Autodesk Inventor part; units mm, degrees
(part 2 of 2)
  spline S141 degree 2 poles (-52.2442, -8.1666) (-52.2404, -7.8589) (-52.0134, -7.5935) (-51.8404, -7.5974) knots 0 0 0 1 2 2 2
  spline S142 degree 2 poles (-51.8404, -7.5974) (-51.675, -7.5935) (-51.4904, -7.8474) (-51.4904, -8.1358) knots 0 0 0 1 2 2 2
  line L206 (-51.4904, -8.1358) -> (-51.4904, -9.6935)
  line L207 (-51.4904, -9.6935) -> (-50.198, -9.6935)
  line L208 (-50.198, -9.6935) -> (-50.198, -8.1666)
  spline S143 degree 2 poles (-50.198, -8.1666) (-50.1942, -7.8589) (-49.9711, -7.5935) (-49.7942, -7.5974) knots 0 0 0 1 2 2 2
  spline S144 degree 2 poles (-49.7942, -7.5974) (-49.6404, -7.5935) (-49.448, -7.8474) (-49.448, -8.1358) knots 0 0 0 1 2 2 2
  line L209 (-49.448, -8.1358) -> (-49.448, -9.6935)
  line L210 (-49.448, -9.6935) -> (-48.1557, -9.6935)
  line L211 (-48.1557, -9.6935) -> (-48.1557, -7.9127)
  spline S145 degree 2 poles (-48.1557, -7.9127) (-48.1596, -7.4204) (-48.4827, -6.8051) (-49.0442, -6.5127) (-49.4019, -6.5127) knots 0 0 0 1 2 3 3 3
  spline S146 degree 2 poles (-45.9442, -9.7512) (-45.4096, -9.7474) (-44.5942, -9.3358) (-44.1327, -8.6089) (-44.1288, -8.1281) knots 0 0 0 1 2 3 3 3
  spline S147 degree 2 poles (-44.1288, -8.1281) (-44.1327, -7.6512) (-44.5942, -6.9243) (-45.4096, -6.5166) (-45.9442, -6.5127) knots 0 0 0 1 2 3 3 3
  spline S148 degree 2 poles (-45.9442, -6.5127) (-46.4788, -6.5166) (-47.2942, -6.9243) (-47.7596, -7.6512) (-47.7634, -8.1281) knots 0 0 0 1 2 3 3 3
  spline S149 degree 2 poles (-47.7634, -8.1281) (-47.7596, -8.6089) (-47.2942, -9.3358) (-46.4788, -9.7474) (-45.9442, -9.7512) knots 0 0 0 1 2 3 3 3
  spline S150 degree 2 poles (-45.9442, -8.7474) (-46.1673, -8.7474) (-46.4519, -8.4358) (-46.4557, -8.1281) knots 0 0 0 1 2 2 2
  spline S151 degree 2 poles (-46.4557, -8.1281) (-46.4519, -7.8243) (-46.1673, -7.5166) (-45.9442, -7.5166) knots 0 0 0 1 2 2 2
  spline S152 degree 2 poles (-45.9442, -7.5166) (-45.725, -7.5166) (-45.4404, -7.8243) (-45.4365, -8.1281) knots 0 0 0 1 2 2 2
  spline S153 degree 2 poles (-45.4365, -8.1281) (-45.4404, -8.4358) (-45.725, -8.7474) (-45.9442, -8.7474) knots 0 0 0 1 2 2 2
  spline S154 degree 2 poles (-40.4865, -7.6051) (-40.2134, -7.4666) (-39.9327, -7.0204) (-39.9327, -6.7397) knots 0 0 0 1 2 2 2
  spline S155 degree 2 poles (-39.9327, -6.7397) (-39.9288, -6.2743) (-40.725, -5.7012) (-41.548, -5.6935) knots 0 0 0 1 2 2 2
  line L212 (-41.548, -5.6935) -> (-43.6865, -5.6935)
  line L213 (-43.6865, -5.6935) -> (-43.6865, -9.6935)
  line L214 (-43.6865, -9.6935) -> (-41.4327, -9.6935)
  spline S156 degree 2 poles (-41.4327, -9.6935) (-40.6057, -9.6897) (-39.748, -9.1166) (-39.7442, -8.5935) knots 0 0 0 1 2 2 2
  spline S157 degree 2 poles (-39.7442, -8.5935) (-39.748, -8.2358) (-40.1327, -7.732) (-40.4865, -7.6051) knots 0 0 0 1 2 2 2
  line L215 (-41.548, -8.7512) -> (-42.3596, -8.7512)
  line L216 (-42.3596, -8.7512) -> (-42.3596, -8.1243)
  line L217 (-42.3596, -8.1243) -> (-41.548, -8.1243)
  spline S158 degree 2 poles (-41.548, -8.1243) (-41.325, -8.1243) (-41.1019, -8.282) (-41.1019, -8.4358) knots 0 0 0 1 2 2 2
  spline S159 degree 2 poles (-41.1019, -8.4358) (-41.1019, -8.5935) (-41.325, -8.7512) (-41.548, -8.7512) knots 0 0 0 1 2 2 2
  spline S160 degree 2 poles (-41.7327, -6.6358) (-41.5057, -6.6358) (-41.2904, -6.7858) (-41.2904, -6.9358) knots 0 0 0 1 2 2 2
  spline S161 degree 2 poles (-41.2904, -6.9358) (-41.2904, -7.082) (-41.5057, -7.232) (-41.7327, -7.232) knots 0 0 0 1 2 2 2
  line L218 (-41.7327, -7.232) -> (-42.3596, -7.232)
  line L219 (-42.3596, -7.232) -> (-42.3596, -6.6358)
  line L220 (-42.3596, -6.6358) -> (-41.7327, -6.6358)
  line L221 (-37.1827, -6.5704) -> (-37.1827, -8.0397)
  spline S162 degree 2 poles (-37.1827, -8.0397) (-37.1904, -8.382) (-37.448, -8.6704) (-37.6211, -8.6666) knots 0 0 0 1 2 2 2
  spline S163 degree 2 poles (-37.6211, -8.6666) (-37.8134, -8.6704) (-38.0288, -8.4012) (-38.0288, -8.0743) knots 0 0 0 1 2 2 2
  line L222 (-38.0288, -8.0743) -> (-38.0288, -6.5704)
  line L223 (-38.0288, -6.5704) -> (-39.3211, -6.5704)
  line L224 (-39.3211, -6.5704) -> (-39.3211, -8.2974)
  spline S164 degree 2 poles (-39.3211, -8.2974) (-39.3173, -8.8012) (-38.975, -9.4474) (-38.3827, -9.7512) (-38.0057, -9.7512) knots 0 0 0 1 2 3 3 3
  spline S165 degree 2 poles (-38.0057, -9.7512) (-37.7519, -9.7512) (-37.298, -9.5781) (-37.1211, -9.3974) knots 0 0 0 1 2 2 2
  line L225 (-37.1211, -9.3974) -> (-37.1211, -9.6935)
  line L226 (-37.1211, -9.6935) -> (-35.8904, -9.6935)
  line L227 (-35.8904, -9.6935) -> (-35.8904, -6.5704)
  line L228 (-35.8904, -6.5704) -> (-37.1827, -6.5704)
  line L229 (-33.1557, -5.4551) -> (-33.1557, -6.782)
  spline S166 degree 2 poles (-33.1557, -6.782) (-33.298, -6.6435) (-33.6904, -6.5127) (-33.948, -6.5127) knots 0 0 0 1 2 2 2
  spline S167 degree 2 poles (-33.948, -6.5127) (-34.3634, -6.5166) (-35.0404, -6.9012) (-35.4519, -7.6243) (-35.4557, -8.1281) knots 0 0 0 1 2 3 3 3
  spline S168 degree 2 poles (-35.4557, -8.1281) (-35.4519, -8.632) (-35.0404, -9.3589) (-34.3634, -9.7474) (-33.948, -9.7512) knots 0 0 0 1 2 3 3 3
  spline S169 degree 2 poles (-33.948, -9.7512) (-33.6596, -9.7512) (-33.2327, -9.5974) (-33.0942, -9.4358) knots 0 0 0 1 2 2 2
  line L230 (-33.0942, -9.4358) -> (-33.0942, -9.6935)
  line L231 (-33.0942, -9.6935) -> (-31.8634, -9.6935)
  line L232 (-31.8634, -9.6935) -> (-31.8634, -5.4551)
  line L233 (-31.8634, -5.4551) -> (-33.1557, -5.4551)
  spline S170 degree 2 poles (-33.6404, -8.7435) (-33.8596, -8.7435) (-34.1442, -8.432) (-34.148, -8.1281) knots 0 0 0 1 2 2 2
  spline S171 degree 2 poles (-34.148, -8.1281) (-34.1442, -7.8243) (-33.8596, -7.5166) (-33.6404, -7.5166) knots 0 0 0 1 2 2 2
  spline S172 degree 2 poles (-33.6404, -7.5166) (-33.4211, -7.5166) (-33.1365, -7.8243) (-33.1327, -8.1281) knots 0 0 0 1 2 2 2
  spline S173 degree 2 poles (-33.1327, -8.1281) (-33.1365, -8.432) (-33.4211, -8.7435) (-33.6404, -8.7435) knots 0 0 0 1 2 2 2
  line L234 (-29.1288, -5.4551) -> (-29.1288, -6.782)
  spline S174 degree 2 poles (-29.1288, -6.782) (-29.2711, -6.6435) (-29.6634, -6.5127) (-29.9211, -6.5127) knots 0 0 0 1 2 2 2
  spline S175 degree 2 poles (-29.9211, -6.5127) (-30.3365, -6.5166) (-31.0134, -6.9012) (-31.425, -7.6243) (-31.4288, -8.1281) knots 0 0 0 1 2 3 3 3
  spline S176 degree 2 poles (-31.4288, -8.1281) (-31.425, -8.632) (-31.0134, -9.3589) (-30.3365, -9.7474) (-29.9211, -9.7512) knots 0 0 0 1 2 3 3 3
  spline S177 degree 2 poles (-29.9211, -9.7512) (-29.6327, -9.7512) (-29.2057, -9.5974) (-29.0673, -9.4358) knots 0 0 0 1 2 2 2
  line L235 (-29.0673, -9.4358) -> (-29.0673, -9.6935)
  line L236 (-29.0673, -9.6935) -> (-27.8365, -9.6935)
  line L237 (-27.8365, -9.6935) -> (-27.8365, -5.4551)
  line L238 (-27.8365, -5.4551) -> (-29.1288, -5.4551)
  spline S178 degree 2 poles (-29.6134, -8.7435) (-29.8327, -8.7435) (-30.1173, -8.432) (-30.1211, -8.1281) knots 0 0 0 1 2 2 2
  spline S179 degree 2 poles (-30.1211, -8.1281) (-30.1173, -7.8243) (-29.8327, -7.5166) (-29.6134, -7.5166) knots 0 0 0 1 2 2 2
  spline S180 degree 2 poles (-29.6134, -7.5166) (-29.3942, -7.5166) (-29.1096, -7.8243) (-29.1057, -8.1281) knots 0 0 0 1 2 2 2
  spline S181 degree 2 poles (-29.1057, -8.1281) (-29.1096, -8.432) (-29.3942, -8.7435) (-29.6134, -8.7435) knots 0 0 0 1 2 2 2
  line L239 (-25.0096, -6.5704) -> (-25.6673, -8.2435)
  line L240 (-25.6673, -8.2435) -> (-26.3096, -6.5704)
  line L241 (-26.3096, -6.5704) -> (-27.6365, -6.5704)
  line L242 (-27.6365, -6.5704) -> (-26.3211, -9.7358)
  spline S182 degree 2 poles (-26.3211, -9.7358) (-26.375, -9.7935) (-26.5288, -9.8589) (-26.6442, -9.8589) knots 0 0 0 1 2 2 2
  spline S183 degree 2 poles (-26.6442, -9.8589) (-26.7596, -9.8589) (-27.0019, -9.7704) (-27.098, -9.6974) knots 0 0 0 1 2 2 2
  line L243 (-27.098, -9.6974) -> (-27.5288, -10.5781)
  spline S184 degree 2 poles (-27.5288, -10.5781) (-27.3634, -10.7089) (-26.8442, -10.8589) (-26.5788, -10.8589) knots 0 0 0 1 2 2 2
  spline S185 degree 2 poles (-26.5788, -10.8589) (-26.248, -10.8627) (-25.6942, -10.6627) (-25.2442, -10.182) (-25.0711, -9.7589) knots 0 0 0 1 2 3 3 3
  line L244 (-25.0711, -9.7589) -> (-23.7865, -6.5704)
  line L245 (-23.7865, -6.5704) -> (-25.0096, -6.5704)
  line L246 (24.7318, 2.5001) -> (24.0485, 3.4796)
  spline S186 degree 2 poles (24.0485, 3.4796) (24.3476, 3.6086) (24.6732, 4.0984) (24.6761, 4.4415) knots 0 0 0 1 2 2 2
  spline S187 degree 2 poles (24.6761, 4.4415) (24.6702, 4.9606) (23.9693, 5.5442) (23.3505, 5.5501) knots 0 0 0 1 2 2 2
  line L247 (23.3505, 5.5501) -> (22.0308, 5.5501)
  line L248 (22.0308, 5.5501) -> (22.0308, 2.5001)
  line L249 (22.0308, 2.5001) -> (22.7376, 2.5001)
  line L250 (22.7376, 2.5001) -> (22.7376, 3.3476)
  line L251 (22.7376, 3.3476) -> (23.3505, 3.3476)
  line L252 (23.3505, 3.3476) -> (23.3857, 3.3476)
  line L253 (23.3857, 3.3476) -> (23.9752, 2.5001)
  line L254 (23.9752, 2.5001) -> (24.7318, 2.5001)
  spline S188 degree 2 poles (23.9605, 4.4415) (23.9605, 4.1923) (23.635, 3.9136) (23.3124, 3.9107) knots 0 0 0 1 2 2 2
  line L255 (23.3124, 3.9107) -> (22.7376, 3.9107)
  line L256 (22.7376, 3.9107) -> (22.7376, 4.9753)
  line L257 (22.7376, 4.9753) -> (23.3124, 4.9753)
  spline S189 degree 2 poles (23.3124, 4.9753) (23.635, 4.9724) (23.9605, 4.6967) (23.9605, 4.4415) knots 0 0 0 1 2 2 2
  line L258 (26.8639, 4.8433) -> (26.8639, 3.682)
  spline S190 degree 2 poles (26.8639, 3.682) (26.8609, 3.3594) (26.5647, 3.0514) (26.3243, 3.0514) knots 0 0 0 1 2 2 2
  spline S191 degree 2 poles (26.3243, 3.0514) (26.0955, 3.0485) (25.8492, 3.3242) (25.8492, 3.6174) knots 0 0 0 1 2 2 2
  line L259 (25.8492, 3.6174) -> (25.8492, 4.8433)
  line L260 (25.8492, 4.8433) -> (25.1688, 4.8433)
  line L261 (25.1688, 4.8433) -> (25.1688, 3.5177)
  spline S192 degree 2 poles (25.1688, 3.5177) (25.1717, 3.157) (25.4239, 2.6907) (25.8756, 2.4649) (26.1718, 2.4649) knots 0 0 0 1 2 3 3 3
  spline S193 degree 2 poles (26.1718, 2.4649) (26.3888, 2.4649) (26.7642, 2.6233) (26.8991, 2.7787) knots 0 0 0 1 2 2 2
  line L262 (26.8991, 2.7787) -> (26.8991, 2.5001)
  line L263 (26.8991, 2.5001) -> (27.5443, 2.5001)
  line L264 (27.5443, 2.5001) -> (27.5443, 4.8433)
  line L265 (27.5443, 4.8433) -> (26.8639, 4.8433)
  spline S194 degree 2 poles (29.6001, 4.8785) (29.3596, 4.8785) (28.9637, 4.7201) (28.8229, 4.5706) knots 0 0 0 1 2 2 2
  line L266 (28.8229, 4.5706) -> (28.8229, 4.8433)
  line L267 (28.8229, 4.8433) -> (28.1748, 4.8433)
  line L268 (28.1748, 4.8433) -> (28.1748, 2.5001)
  line L269 (28.1748, 2.5001) -> (28.8552, 2.5001)
  line L270 (28.8552, 2.5001) -> (28.8552, 3.6585)
  spline S195 degree 2 poles (28.8552, 3.6585) (28.8581, 3.9811) (29.166, 4.292) (29.4153, 4.292) knots 0 0 0 1 2 2 2
  spline S196 degree 2 poles (29.4153, 4.292) (29.6441, 4.292) (29.8904, 4.0222) (29.8904, 3.7377) knots 0 0 0 1 2 2 2
  line L271 (29.8904, 3.7377) -> (29.8904, 2.5001)
  line L272 (29.8904, 2.5001) -> (30.5708, 2.5001)
  line L273 (30.5708, 2.5001) -> (30.5708, 3.8433)
  spline S197 degree 2 poles (30.5708, 3.8433) (30.5679, 4.1981) (30.3157, 4.6586) (29.8787, 4.8785) (29.6001, 4.8785) knots 0 0 0 1 2 3 3 3
  line L274 (23.3505, 14.5501) -> (22.0308, 14.5501)
  line L275 (22.0308, 14.5501) -> (22.0308, 11.5001)
  line L276 (22.0308, 11.5001) -> (22.7376, 11.5001)
  line L277 (22.7376, 11.5001) -> (22.7376, 12.3418)
  line L278 (22.7376, 12.3418) -> (23.3505, 12.3418)
  spline S198 degree 2 poles (23.3505, 12.3418) (23.9693, 12.3476) (24.6702, 12.9283) (24.6761, 13.4445) knots 0 0 0 1 2 2 2
  spline S199 degree 2 poles (24.6761, 13.4445) (24.6702, 13.9606) (23.9693, 14.5442) (23.3505, 14.5501) knots 0 0 0 1 2 2 2
  line L279 (23.3124, 12.9166) -> (22.7376, 12.9166)
  line L280 (22.7376, 12.9166) -> (22.7376, 13.9753)
  line L281 (22.7376, 13.9753) -> (23.3124, 13.9753)
  spline S200 degree 2 poles (23.3124, 13.9753) (23.635, 13.9724) (23.9605, 13.6967) (23.9605, 13.4445) knots 0 0 0 1 2 2 2
  spline S201 degree 2 poles (23.9605, 13.4445) (23.9605, 13.1923) (23.635, 12.9195) (23.3124, 12.9166) knots 0 0 0 1 2 2 2
  spline S202 degree 2 poles (26.2861, 11.4649) (26.6615, 11.4678) (27.2393, 11.7728) (27.5677, 12.3154) (27.5707, 12.6732) knots 0 0 0 1 2 3 3 3
  spline S203 degree 2 poles (27.5707, 12.6732) (27.5677, 13.028) (27.2393, 13.5706) (26.6615, 13.8756) (26.2861, 13.8785) knots 0 0 0 1 2 3 3 3
  spline S204 degree 2 poles (26.2861, 13.8785) (25.9107, 13.8756) (25.3301, 13.5706) (24.9987, 13.028) (24.9957, 12.6732) knots 0 0 0 1 2 3 3 3
  spline S205 degree 2 poles (24.9957, 12.6732) (24.9987, 12.3154) (25.3301, 11.7728) (25.9107, 11.4678) (26.2861, 11.4649) knots 0 0 0 1 2 3 3 3
  spline S206 degree 2 poles (26.2861, 12.0221) (26.0251, 12.025) (25.6908, 12.3652) (25.6849, 12.6732) knots 0 0 0 1 2 2 2
  spline S207 degree 2 poles (25.6849, 12.6732) (25.6908, 12.9782) (26.0251, 13.3184) (26.2861, 13.3213) knots 0 0 0 1 2 2 2
  spline S208 degree 2 poles (26.2861, 13.3213) (26.5442, 13.3184) (26.8756, 12.9782) (26.8815, 12.6732) knots 0 0 0 1 2 2 2
  spline S209 degree 2 poles (26.8815, 12.6732) (26.8756, 12.3652) (26.5442, 12.025) (26.2861, 12.0221) knots 0 0 0 1 2 2 2
  line L282 (31.1867, 13.8433) -> (30.6148, 12.2567)
  line L283 (30.6148, 12.2567) -> (30.0576, 13.8433)
  line L284 (30.0576, 13.8433) -> (29.4828, 13.8433)
  line L285 (29.4828, 13.8433) -> (28.908, 12.2567)
  line L286 (28.908, 12.2567) -> (28.3537, 13.8433)
  line L287 (28.3537, 13.8433) -> (27.7144, 13.8433)
  line L288 (27.7144, 13.8433) -> (28.559, 11.5001)
  line L289 (28.559, 11.5001) -> (29.213, 11.5001)
  line L290 (29.213, 11.5001) -> (29.7584, 12.9547)
  line L291 (29.7584, 12.9547) -> (30.2834, 11.5001)
  line L292 (30.2834, 11.5001) -> (30.9374, 11.5001)
  line L293 (30.9374, 11.5001) -> (31.7879, 13.8433)
  line L294 (31.7879, 13.8433) -> (31.1867, 13.8433)
  spline S210 degree 2 poles (34.4009, 12.6614) (34.398, 13.0427) (34.0783, 13.5852) (33.5299, 13.8756) (33.1809, 13.8785) knots 0 0 0 1 2 3 3 3
  spline S211 degree 2 poles (33.1809, 13.8785) (32.8202, 13.8756) (32.26, 13.5676) (31.9345, 13.0251) (31.9316, 12.6702) knots 0 0 0 1 2 3 3 3
  spline S212 degree 2 poles (31.9316, 12.6702) (31.9345, 12.3212) (32.263, 11.7787) (32.8612, 11.4678) (33.2689, 11.4649) knots 0 0 0 1 2 3 3 3
  spline S213 degree 2 poles (33.2689, 11.4649) (33.5856, 11.4649) (34.0724, 11.6585) (34.2367, 11.8432) knots 0 0 0 1 2 2 2
  line L295 (34.2367, 11.8432) -> (33.873, 12.2362)
  spline S214 degree 2 poles (33.873, 12.2362) (33.7557, 12.1218) (33.4712, 12.0104) (33.2865, 12.0104) knots 0 0 0 1 2 2 2
  spline S215 degree 2 poles (33.2865, 12.0104) (33.0167, 12.0133) (32.6677, 12.2597) (32.6149, 12.4796) knots 0 0 0 1 2 2 2
  line L296 (32.6149, 12.4796) -> (34.3862, 12.4796)
  spline S216 degree 2 poles (34.3862, 12.4796) (34.3921, 12.5236) (34.4009, 12.6233) (34.4009, 12.6614) knots 0 0 0 1 2 2 2
  spline S217 degree 2 poles (33.1868, 13.3653) (33.4184, 13.3624) (33.7205, 13.1013) (33.7616, 12.8755) knots 0 0 0 1 2 2 2
  line L297 (33.7616, 12.8755) -> (32.6061, 12.8755)
  spline S218 degree 2 poles (32.6061, 12.8755) (32.6442, 13.1043) (32.9521, 13.3624) (33.1868, 13.3653) knots 0 0 0 1 2 2 2
  line L298 (35.5007, 13.5354) -> (35.5007, 13.8433)
  line L299 (35.5007, 13.8433) -> (34.8525, 13.8433)
  line L300 (34.8525, 13.8433) -> (34.8525, 11.5001)
  line L301 (34.8525, 11.5001) -> (35.5329, 11.5001)
  line L302 (35.5329, 11.5001) -> (35.5329, 12.6057)
  spline S219 degree 2 poles (35.5329, 12.6057) (35.5358, 12.943) (35.8702, 13.2597) (36.1546, 13.2597) knots 0 0 0 1 2 2 2
  spline S220 degree 2 poles (36.1546, 13.2597) (36.1928, 13.2597) (36.2661, 13.2538) (36.3071, 13.2509) knots 0 0 0 1 2 2 2
  line L303 (36.3071, 13.2509) -> (36.3071, 13.8785)
  spline S221 degree 2 poles (36.3071, 13.8785) (36.0344, 13.8785) (35.6268, 13.7055) (35.5007, 13.5354) knots 0 0 0 1 2 2 2
  point P0 (0, 0)
  point P1 (-52.241, -25.46)
  point P2 (-12.021, -25.46)
  point P3 (-56.021, -25.46)
  point P4 (-68.241, -25.46)
  dimension "d70" = 4
  dimension "d71" = 1
  dimension "d72" = 0.4
  dimension "d75" = 5
  constraints: 60 end point, 18 horizontal, 15 vertical alignment, 10 parallel, 8 point on line, 6 collinear, 6 midpoint, 6 perpendicular, 2 coincident, 1 vertical, 4 other
  measures "d70" distance of L1.start L0.start
  measures "d71" distance between parallel lines of L19 L17
  measures "d72" distance between parallel lines of L17 L7
  measures "d75" distance of L43.start L43.end
extrude "Extrusion14" cut sketch "Sketch14" against normal blind 0.0001
body "Solid1"
